Autodesk Fusion 360 part; units mm, degrees
(part 2 of 2)
sketch "sketch 3678" plane through (0, 0, 1) normal (0, 0, 1) x (-1, 0, 0)
  line L0 (-70.1201, -10.426) -> (-62.6519, -10.426)
  line L1 (-70.1201, -11.607) -> (-70.1201, -10.426)
  line L2 (-63.9763, -11.607) -> (-70.1201, -11.607)
  line L3 (-63.9763, -15.0134) -> (-63.9763, -11.607)
  line L4 (-69.5125, -15.0134) -> (-63.9763, -15.0134)
  line L5 (-69.5125, -16.1876) -> (-69.5125, -15.0134)
  line L6 (-63.9763, -16.1876) -> (-69.5125, -16.1876)
  line L7 (-63.9763, -19.2526) -> (-63.9763, -16.1876)
  line L8 (-69.888, -19.2526) -> (-63.9763, -19.2526)
  line L9 (-69.888, -20.4336) -> (-69.888, -19.2526)
  line L10 (-62.6519, -20.4336) -> (-69.888, -20.4336)
  line L11 (-62.6519, -10.426) -> (-62.6519, -20.4336)
  line L12 (-55.45, -19.1229) -> (-50.5486, -19.1229)
  spline S0 degree 3 poles (-53.6854, -16.505) (-53.9568, -16.9914) (-54.4716, -17.9139) (-55.136, -18.7349) (-55.45, -19.1229) knots 0 0 0 0 0.166741 0.316231 0.316231 0.316231 0.316231
  spline S1 degree 3 poles (-52.4122, -13.2795) (-52.5768, -13.8331) (-52.9074, -14.9453) (-53.4253, -15.9836) (-53.6854, -16.505) knots 0 0 0 0 0.172915 0.347351 0.347351 0.347351 0.347351
  spline S2 degree 3 poles (-51.948, -10.426) (-51.9786, -10.8625) (-52.0462, -11.8273) (-52.2827, -12.7656) (-52.4122, -13.2795) knots 0 0 0 0 0.130996 0.289598 0.289598 0.289598 0.289598
  line L13 (-53.2109, -10.426) -> (-51.948, -10.426)
  spline S3 degree 3 poles (-53.682, -13.1771) (-53.5697, -12.7405) (-53.3372, -11.8366) (-53.254, -10.9068) (-53.2109, -10.426) knots 0 0 0 0 0.135003 0.27952 0.27952 0.27952 0.27952
  spline S4 degree 3 poles (-55.1326, -16.6449) (-54.8384, -16.082) (-54.2559, -14.9674) (-53.872, -13.7698) (-53.682, -13.1771) knots 0 0 0 0 0.190168 0.376518 0.376518 0.376518 0.376518
  spline S5 degree 3 poles (-57.0269, -19.3482) (-56.6983, -18.9616) (-55.9829, -18.1199) (-55.431, -17.1625) (-55.1326, -16.6449) knots 0 0 0 0 0.151922 0.330698 0.330698 0.330698 0.330698
  line L14 (-57.0269, -20.3039) -> (-57.0269, -19.3482)
  line L15 (-50.5486, -20.3039) -> (-57.0269, -20.3039)
  line L16 (-50.5486, -19.1229) -> (-50.5486, -20.3039)
extrude "Extrude1" add sketch "Sketch1" sketch "sketch 2408" sketch "sketch 2641" sketch "sketch 2864" sketch "sketch 3108" sketch "sketch 3361" sketch "sketch 3572" sketch "sketch 3678" along normal blind 0.5 of sketch 2 of sketch 3 of sketch 4 of sketch 5 of sketch 6 of sketch 7 of sketch 8 makes body 1 at (88.4257, 31.9948, 1) makes body 2 at (169.2987, 38.6685, 1) makes body 3 at (-21.6109, 38.9553, 1) makes body 4 at (131.1987, 38.6685, 1) makes body 5 at (202.7257, 31.9948, 1) makes body 6 at (16.4891, 38.9553, 1) makes body 7 at (54.9987, 38.6685, 1) makes body 8 at (24.921, 15.1578, 1) makes body 9 at (-19.2872, 14.9279, 1) makes body 10 at (12.6697, 15.6307, 1) makes body 11 at (54.3419, 19.9103, 1) makes body 12 at (63.0934, 15.291, 1) makes body 13 at (101.733, 15.291, 1) makes body 14 at (93.268, 15.8375, 1) makes body 15 at (139.4742, 15.129, 1) makes body 16 at (133.0011, 14.7659, 1) makes body 17 at (168.7538, 20.2343, 1) makes body 18 at (182.1383, 15.4558, 1) makes body 19 at (207.4843, 15.8375, 1) makes body 20 at (-8.1812, 15.1317, 1) makes body 21 at (220.5821, 15.1317, 1)
